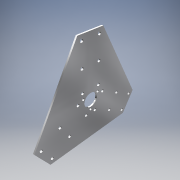
# Autodesk Inventor part: Outer Gusset Plate
Saved by Autodesk Inventor 2019 (Build 230136000, 136)
## iProperties
Created: 2018-09-22
Part Number: Outer Gusset Plate
Material: Aluminum 6061
Document SubType Name: Modeling
Designer: Adhik
Density: 2.7 g/cm^3
Appearance: Aluminum - Flat
Mass: 263.149 g
Surface Area: 651.373 cm^2
Volume: 97.4625 cm^3
Author: Adhik
Autodesk Inventor part; units mm, degrees
ref_plane "YZ Plane" through (0, 0, 0) normal (1, 0, 0) x (0, 1, 0)
ref_plane "XZ Plane" through (0, 0, 0) normal (0, 1, 0) x (-1, 0, 0)
ref_plane "XY Plane" through (0, 0, 0) normal (0, 0, 1) x (1, 0, 0)
sketch "Sketch1" plane through (0, 0, 0) normal (1, 0, 0) x (0, 1, 0)
  line L0 (0, -164.2446) -> (0, 164.2446) construction
  line L1 (-123.038, 0) -> (161.442, 0) construction
  line L2 (120.802, 25.4) -> (120.802, -25.4)
  line L3 (120.802, -25.4) -> (-38.4039, -117.3176)
  line L4 (-38.4039, -117.3176) -> (-82.398, -91.9176)
  line L5 (-82.398, -91.9176) -> (-82.398, 91.9176)
  line L6 (-82.398, 91.9176) -> (-38.4039, 117.3176)
  line L7 (-38.4039, 117.3176) -> (120.802, 25.4)
  line L8 (-60.401, 104.6176) -> (41.199, -71.3588) construction
  line L9 (-40.1887, 105.1689) -> (-70.9846, 87.3889) construction
  line L10 (-70.9846, 87.3889) -> (-26.5346, 10.3993) construction
  line L11 (-26.5346, 10.3993) -> (4.2613, 28.1793) construction
  line L12 (4.2613, 28.1793) -> (-40.1887, 105.1689) construction
  circle A0 centre (-40.1887, 105.1689) radius 3.175
  circle A1 centre (-70.9846, 87.3889) radius 3.175
  circle A2 centre (4.2613, 28.1793) radius 3.175
  circle A3 centre (-26.5346, 10.3993) radius 3.175
  circle A4 centre (-17.9637, 66.6741) radius 3.175
  circle A5 centre (-48.7596, 48.8941) radius 3.175
  line L13 (-38.4039, 117.3176) -> (14.6647, 25.4) construction
  line L14 (14.6647, 25.4) -> (-29.3294, 0) construction
  line L15 (-29.3294, 0) -> (-82.398, 91.9176) construction
  line L16 (-41.1536, 115.7301) -> (11.9151, 23.8125) construction
  circle A6 centre (-70.9846, -87.3889) radius 3.175
  circle A7 centre (-48.7596, -48.8941) radius 3.175
  circle A8 centre (-26.5346, -10.3993) radius 3.175
  circle A9 centre (4.2613, -28.1793) radius 3.175
  circle A10 centre (-17.9637, -66.6741) radius 3.175
  circle A11 centre (-40.1887, -105.1689) radius 3.175
  circle A12 centre (111.1733, -17.78) radius 3.175
  circle A13 centre (66.7233, -17.78) radius 3.175
  circle A14 centre (22.2733, -17.78) radius 3.175
  circle A15 centre (22.2733, 17.78) radius 3.175
  circle A16 centre (66.7233, 17.78) radius 3.175
  circle A17 centre (111.1733, 17.78) radius 3.175
  circle A18 centre (0, 0) radius 14.6647 construction
  circle A19 centre (0, 0) radius 14.2875
  point P0 (120.802, 0)
  point P1 (-82.398, 0)
  point P2 (-55.5867, 96.2789)
  point P3 (-11.1367, 19.2893)
  dimension "d0" = 203.2
  dimension "d1" = 50.8
  dimension "d2" = 6.35
  dimension "d4" = 3.175
  dimension "d7" = 17.78
  dimension "d10" = 360
  dimension "d14" = 29.3294
  dimension "d15" = 28.575
  dimension "d32" = 88.9
  dimension "d33" = 7.6086
  constraints: 30 end point, 20 centre point, 8 midpoint, 8 point on line, 6 coincident, 5 equal radius, 5 parallel, 4 equal length, 4 perpendicular, 1 tangent, 1 vertical, 37 other
  measures "d0" distance between parallel lines of L5 L2
  measures "d1" distance of L2.start L2.end
  measures "d2" diameter of A0
  measures "d4" distance between parallel lines of L13 L16
  measures "d7" distance between parallel lines of L8 L12
  measures "d14" diameter of A18
  measures "d15" diameter of A19
  measures "d32" distance of L11.end L9.start
  measures "d33" distance between parallel lines of L14 L11
extrude "Extrusion2" add sketch "Sketch1" along normal blind 3.175
sketch "Sketch2" plane through (3.175, 0, 0) normal (1, 0, 0) x (0, 0, -1)
  circle A0 centre (0, 0) radius 15.875 construction
  line L0 (164.2446, 0) -> (-164.2446, 0) construction
  line L1 (0, -123.038) -> (0, 161.442) construction
  line L2 (0, 0) -> (-16.4978, 9.525) construction
  circle A1 centre (-16.4978, 9.525) radius 3.175 construction
  circle A2 centre (0, -19.05) radius 3.175 construction
  circle A3 centre (16.4978, 9.525) radius 3.175 construction
  circle A4 centre (-16.4978, 9.525) radius 2.667
  circle A5 centre (0, -19.05) radius 2.667
  circle A6 centre (16.4978, 9.525) radius 2.667
  dimension "d18" = 31.75
  dimension "d19" = 30
  dimension "d20" = 6.35
  dimension "d23" = 360
  dimension "d25" = 5.334
  dimension "d28" = 360
  constraints: 7 centre point, 3 coincident, 2 end point, 1 tangent, 14 other
  measures "d18" diameter of A0
  measures "d19" angle of L0 L2
  measures "d20" diameter of A1
  measures "d25" diameter of A4
extrude "Extrusion3" cut sketch "Sketch2" against normal through all
sketch "Sketch3" plane through (3.175, 0, 0) normal (1, 0, 0) x (0, 0, -1)
  line L0 (0, -123.038) -> (0, 161.442) construction
  line L1 (164.2446, 0) -> (-164.2446, 0) construction
  line L2 (-91.9176, -82.398) -> (0, -29.3294) construction
  line L3 (0, -29.3294) -> (91.9176, -82.398) construction
  line L4 (-117.3176, -38.4039) -> (-91.9176, -82.398) construction
  line L5 (-91.9176, -82.398) -> (91.9176, -82.398) construction
  line L6 (-74.5691, -76.048) -> (-55.3084, -64.9279)
  line L7 (-55.3084, -64.9279) -> (-48.8882, -76.048)
  line L8 (-48.8882, -76.048) -> (-74.5691, -76.048)
  line L9 (-3.175, -76.048) -> (-21.0235, -45.1335)
  line L10 (-21.0235, -45.1335) -> (-3.175, -34.8287)
  line L11 (-3.175, -34.8287) -> (-3.175, -76.048)
  line L12 (-43.3889, -72.873) -> (-49.8092, -61.7529)
  line L13 (-49.8092, -61.7529) -> (-30.5485, -50.6328)
  line L14 (-30.5485, -50.6328) -> (-43.3889, -72.873)
  line L15 (-24.1985, -52.3342) -> (-37.8897, -76.048)
  line L16 (-37.8897, -76.048) -> (-10.5073, -76.048)
  line L17 (-10.5073, -76.048) -> (-24.1985, -52.3342)
  line L18 (-48.8882, -76.048) -> (-37.8897, -76.048) construction
  line L19 (-30.5485, -50.6328) -> (-21.0235, -45.1335) construction
  line L20 (74.5691, -76.048) -> (55.3084, -64.9279)
  line L21 (55.3084, -64.9279) -> (48.8882, -76.048)
  line L22 (48.8882, -76.048) -> (74.5691, -76.048)
  line L23 (3.175, -76.048) -> (21.0235, -45.1335)
  line L24 (21.0235, -45.1335) -> (3.175, -34.8287)
  line L25 (3.175, -34.8287) -> (3.175, -76.048)
  line L26 (43.3889, -72.873) -> (49.8092, -61.7529)
  line L27 (49.8092, -61.7529) -> (30.5485, -50.6328)
  line L28 (30.5485, -50.6328) -> (43.3889, -72.873)
  line L29 (24.1985, -52.3342) -> (37.8897, -76.048)
  line L30 (37.8897, -76.048) -> (10.5073, -76.048)
  line L31 (10.5073, -76.048) -> (24.1985, -52.3342)
  point P0 (0, 0)
  dimension "d34" = 3.175
  dimension "d35" = 6.35
  dimension "d36" = 3.175
  dimension "d37" = 6.35
  dimension "d38" = 6.35
  dimension "d39" = 6.35
  constraints: 58 end point, 12 symmetric about line, 4 equal length, 4 parallel, 3 collinear, 3 horizontal, 3 perpendicular, 3 point on line, 1 coincident, 1 vertical, 1 other
  measures "d34" distance between parallel lines of L2 L6
  measures "d35" distance between parallel lines of L5 L8
  measures "d36" distance between parallel lines of L0 L11
  measures "d37" distance between parallel lines of L12 L7
  measures "d38" distance between parallel lines of L14 L15
  measures "d39" distance between parallel lines of L9 L17
extrude "Extrusion4" [suppressed]
chamfer "Chamfer1" [suppressed]
fillet "Fillet1" [suppressed]
pattern_circular "Circular Pattern1" [suppressed]
equation "\"d36\" = 0.5 * d35"
equation "\"d37\" = d35"
equation "\"d38\" = d35"
equation "\"d39\" = d35"
body "Solid2"
